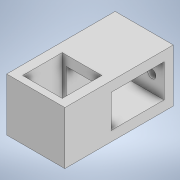
# Autodesk Inventor part: loacell_mount1
Saved by Autodesk Inventor 2022.3 (Build 263350000, 350)
## iProperties
Created: 2022-06-09
Part Number: loacell_mount1
Material: Generic
Document SubType Name: Modeling
Designer: Martijn
Density: 1 g/cm^3
Appearance: Default
Author: Martijn
Autodesk Inventor part; units mm, degrees
ref_plane "YZ Plane" through (0, 0, 0) normal (1, 0, 0) x (0, 1, 0)
ref_plane "XZ Plane" through (0, 0, 0) normal (0, 1, 0) x (-1, 0, 0)
ref_plane "XY Plane" through (0, 0, 0) normal (0, 0, 1) x (1, 0, 0)
sketch "Sketch1" plane through (0, 0, 0) normal (0, 0, 1) x (1, 0, 0)
  line L0 (0, 0) -> (44, 0)
  line L1 (44, 0) -> (44, 40)
  line L2 (44, 40) -> (0, 40)
  line L3 (0, 40) -> (0, 0)
  dimension "d0" = 44
  dimension "d1" = 40
  constraints: 8 end point, 2 parallel, 1 horizontal, 1 perpendicular
  measures "d0" distance of L0.start L0.end
  measures "d1" distance of L2.end L0.start
extrude "Extrusion1" add sketch "Sketch1" along normal blind 82
sketch "Sketch2" plane through (0, 0, 0) normal (0, -1, 0) x (1, 0, 0)
  line L0 (7, 77) -> (37, 77)
  line L1 (37, 77) -> (37, 47)
  line L2 (37, 47) -> (7, 47)
  line L3 (7, 47) -> (7, 77)
  line L4 (0, 0) -> (0, 82) projected
  line L5 (0, 82) -> (44, 82) projected
  dimension "d4" = 30
  dimension "d5" = 30
  dimension "d6" = 7
  dimension "d7" = 5
  constraints: 8 end point, 2 parallel, 1 horizontal, 1 perpendicular
  measures "d4" distance of L0.start L0.end
  measures "d5" distance of L2.end L0.start
  measures "d6" distance between parallel lines of L4 L3
  measures "d7" distance between parallel lines of L5 L0
extrude "Extrusion2" cut sketch "Sketch2" against normal blind 50
sketch "Sketch4" plane through (44, 0, 0) normal (1, 0, 0) x (0, 0, -1)
  line L0 (-7, 7.5) -> (-47, 7.5)
  line L1 (-47, 7.5) -> (-47, 32.5)
  line L2 (-47, 32.5) -> (-7, 32.5)
  line L3 (-7, 32.5) -> (-7, 7.5)
  line L4 (0, 0) -> (0, 40) projected
  line L5 (0, 0) -> (-82, 0) projected
  line L6 (-47, 0) -> (-47, 40) projected
  point P0 (0, 20)
  point P1 (-7, 20)
  dimension "d10" = 25
  dimension "d11" = 40
  dimension "d13" = 7.5
  constraints: 8 end point, 2 midpoint, 2 parallel, 1 collinear, 1 horizontal, 1 perpendicular
  measures "d10" distance between parallel lines of L0 L2
  measures "d11" distance between parallel lines of L3 L1
  measures "d13" distance between parallel lines of L5 L0
extrude "Extrusion3" cut sketch "Sketch4" against normal blind 34
sketch "Sketch5" plane through (0, 0, 0) normal (0, 0, -1) x (-1, 0, 0)
  circle A0 centre (-15.8, 20) radius 3.1
  circle A1 centre (-34.8, 20) radius 3.1
  line L0 (-44, 40) -> (0, 40) projected
  line L1 (-10, 7.5) -> (-10, 32.5) projected
  point P0 (0, 0)
  dimension "d16" = 6.2
  dimension "d17" = 6.2
  dimension "d18" = 20
  dimension "d19" = 20
  dimension "d20" = 5.8
  dimension "d21" = 19
  constraints: 2 centre point
  measures "d16" diameter of A0
  measures "d17" diameter of A1
  measures "d18" distance from line of L0 A0.centre
  measures "d19" distance from line of L0 A1.centre
  measures "d20" distance from line of L1 A0.centre
  measures "d21" distance of A0.centre A1.centre
extrude "Extrusion4" cut sketch "Sketch5" against normal blind 34
body "Solid1"
